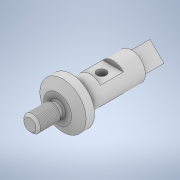
# Autodesk Inventor part: Деталь2
Saved by Autodesk Inventor 2020 (Build 240168000, 168)
## iProperties
Created: 2020-03-27
Part Number: Деталь2
Material: Типовые
Document SubType Name: Modeling
Designer: Trickster2038
Density: 1 g/cm^3
Appearance: По умолчанию
Mass: 81.9997 g
Surface Area: 157.002 cm^2
Volume: 81.9997 cm^3
Author: Trickster2038
Autodesk Inventor part; units mm, degrees
sketch "Эскиз1" plane through (0, 0, 0) normal (0, 0, 1) x (1, 0, 0)
  circle A0 centre (0, 0) radius 9
  constraints: 1 centre point, 1 coincident
sketch "Эскиз2" plane through (0, 0, 0) normal (0, 0, 1) x (1, 0, 0)
  point P0 (0, 0)
extrude "Выдавливание1" add sketch "Эскиз1" along normal blind 30
ref_plane "РабПлоскость1" through (0, 0, 0) normal (0, 0, 1) x (1, 0, 0)
sketch "Эскиз3" plane through (0, 0, 0) normal (0, 0, 1) x (1, 0, 0)
  circle A0 centre (0, 0) radius 25
  constraints: 1 centre point, 1 coincident
extrude "Выдавливание2" add sketch "Эскиз3" against normal blind 15
ref_plane "РабПлоскость2" through (0, 0, -15) normal (0, 0, -1) x (-1, 0, 0)
sketch "Эскиз4" plane through (0, 0, -15) normal (0, 0, -1) x (-1, 0, 0)
  circle A0 centre (0, 0) radius 15
  constraints: 1 centre point, 1 coincident
extrude "Выдавливание3" add sketch "Эскиз4" along normal blind 20
ref_plane "РабПлоскость3" through (0, 0, -35) normal (0, 0, -1) x (-1, 0, 0)
sketch "Эскиз5" plane through (0, 0, -35) normal (0, 0, -1) x (-1, 0, 0)
  circle A0 centre (0, 0) radius 15
  constraints: 1 centre point, 1 coincident
extrude "Выдавливание4" add sketch "Эскиз5" along normal blind 25
ref_plane "РабПлоскость4" through (0, 0, -60) normal (0, 0, -1) x (-1, 0, 0)
sketch "Эскиз6" plane through (0, 0, -60) normal (0, 0, -1) x (-1, 0, 0)
  circle A0 centre (0, 0) radius 9 projected
  circle A1 centre (0, 0) radius 15
  constraints: 1 centre point, 1 coincident
extrude "Выдавливание5" add sketch "Эскиз6" along normal blind 20 contours A0 | A1
ref_plane "РабПлоскость5" through (0, 0, -80) normal (0, 0, -1) x (-1, 0, 0)
sketch "Эскиз7" plane through (0, 0, -80) normal (0, 0, -1) x (-1, 0, 0)
  circle A0 centre (0, 0) radius 15 projected
  line L0 (0, 15) -> (15, 0)
  line L1 (15, 0) -> (0, -15)
  line L2 (0, -15) -> (-15, 0)
  line L3 (-15, 0) -> (0, 15)
  constraints: 8 end point, 1 coincident, 1 vertical alignment, 10 other
extrude "Выдавливание6" add sketch "Эскиз7" along normal blind 20 contours L1 L2 L3 L0
sketch "Эскиз8" plane through (0, 0, 0) normal (1, 0, 0) x (0, 1, 0)
  line L0 (0, 0) -> (0, -35)
  line L1 (0, -35) -> (10, -35)
  line L2 (10, -35) -> (-10, -35)
  line L3 (-10, -35) -> (-10, -60)
  line L4 (-10, -60) -> (-25, -60)
  line L5 (-25, -60) -> (-25, -35)
  line L6 (-25, -35) -> (-10, -35)
  line L7 (10, -35) -> (10, -60)
  line L8 (10, -60) -> (25, -60)
  line L9 (25, -60) -> (25, -35)
  line L10 (25, -35) -> (10, -35)
  dimension "d22" = 35
  dimension "d23" = 10
  dimension "d24" = 20
  dimension "d25" = 25
  dimension "d26" = 15
  dimension "d27" = 15
  constraints: 22 end point, 7 perpendicular, 5 point on line, 1 collinear, 1 vertical
  measures "d22" distance of L0.start L0.end
  measures "d23" distance of L0.end L1.end
  measures "d24" distance of L1.end L2.end
  measures "d25" distance of L2.end L3.end
  measures "d26" distance of L3.end L4.end
  measures "d27" distance of L7.end L8.end
extrude "Выдавливание7" cut sketch "Эскиз8" against normal mid plane 40 contours L10 L9 L8 L7
sketch "Эскиз9" plane through (0, 0, 0) normal (1, 0, 0) x (0, 1, 0)
  line L0 (0, 0) -> (0, -35)
  line L1 (0, -35) -> (-10, -35)
  line L2 (-10, -35) -> (-10, -60)
  line L3 (-10, -60) -> (-25, -60)
  line L4 (-25, -60) -> (-25, -35)
  line L5 (-25, -35) -> (-10, -35)
  dimension "d30" = 35
  dimension "d31" = 10
  dimension "d32" = 25
  dimension "d33" = 15
  constraints: 12 end point, 5 perpendicular, 1 point on line, 1 vertical
  measures "d30" distance of L0.start L0.end
  measures "d31" distance of L0.end L1.end
  measures "d32" distance of L1.end L2.end
  measures "d33" distance of L2.end L3.end
extrude "Выдавливание8" cut sketch "Эскиз9" along normal mid plane 40
sketch "Эскиз10" plane through (0, 0, 0) normal (1, 0, 0) x (0, 1, 0)
  point P0 (0, 0)
sketch "Эскиз11" plane through (0, 0, 0) normal (0, 1, 0) x (-1, 0, 0)
  line L0 (0, 0) -> (0, -47.5)
  circle A0 centre (0, -47.5) radius 5
  dimension "d36" = 47.5
  dimension "d37" = 10
  constraints: 2 end point, 1 centre point, 1 coincident, 1 vertical
  measures "d36" distance of L0.start L0.end
  measures "d37" diameter of A0
extrude "Выдавливание9" cut sketch "Эскиз11" along normal mid plane 40
chamfer "Фаска1" distance 2.5 angle 45 1 edges at (-9, 0, 30)
chamfer "Фаска2" distance 10 angle 30 1 edges at (-25, 0, 0) measured on face at (19.3373, -2.7122, 0)
sketch "Эскиз12" plane through (0, 0, 0) normal (0, 1, 0) x (-1, 0, 0)
  line L0 (0, 0) -> (25, 0)
  line L1 (25, 0) -> (25, 4)
  line L2 (25, 4) -> (25, 6)
  line L3 (25, 6) -> (-25.3406, 6)
  line L4 (-25.3406, 6) -> (-25.3406, 0)
  line L5 (-25.3406, 0) -> (25, 0)
  dimension "d48" = 4
  dimension "d49" = 2
  constraints: 12 end point, 4 perpendicular, 2 point on line, 1 horizontal
  measures "d48" distance of L0.end L1.end
  measures "d49" distance of L1.end L2.end
extrude "Выдавливание10" cut sketch "Эскиз12" against normal mid plane 40
sketch "Эскиз13" plane through (0, 0, 0) normal (0, 0, 1) x (1, 0, 0)
  circle A0 centre (0, 0) radius 7.25
  dimension "d52" = 14.5
  constraints: 1 centre point, 1 coincident
  measures "d52" diameter of A0
extrude "Выдавливание11" add sketch "Эскиз13" along normal blind 6
fillet "Сопряжение1" radius 1 1 edges at (-7.25, 0, 6)
thread "Резьба2" size "M18x1.25" class "6g" standard "ANSI Metric M Profile" length 24
fillet "Сопряжение2" radius 1.6 1 edges at (-7.25, 0, 0)
